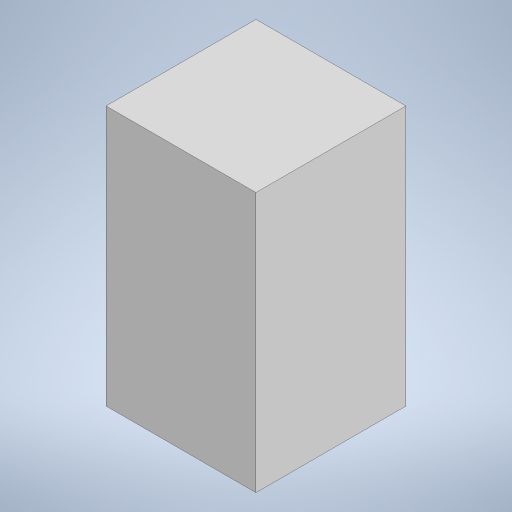
# Autodesk Inventor part: body_luggage
Saved by Autodesk Inventor 2024.3 (Build 283343000, 343)
## iProperties
Created: 2025-04-01
Part Number: body_luggage
Material: 一般
Document SubType Name: Modeling
Designer: yuu53
Density: 1 g/cm^3
Appearance: 既定
Author: yuu53
Autodesk Inventor part; units mm, degrees
ref_plane "YZ Plane" through (0, 0, 0) normal (1, 0, 0) x (0, 1, 0)
ref_plane "XZ Plane" through (0, 0, 0) normal (0, 1, 0) x (-1, 0, 0)
ref_plane "XY Plane" through (0, 0, 0) normal (0, 0, 1) x (1, 0, 0)
sketch "スケッチ1" plane through (0, 0, 0) normal (0, 0, 1) x (1, 0, 0)
  line L0 (-75, -130) -> (75, -130)
  line L1 (75, -130) -> (75, 130)
  line L2 (75, 130) -> (-75, 130)
  line L3 (-75, 130) -> (-75, -130)
  point P0 (0, 0)
  point P1 (75, 0)
  dimension "d0" = 260
  dimension "d1" = 150
  dimension "d3" = 75
  dimension "d4" = 130
  constraints: 8 end point, 2 parallel, 1 horizontal, 1 midpoint, 1 perpendicular
  measures "d0" distance of L0.end L1.end
  measures "d1" distance of L1.end L2.end
  measures "d3" distance from line of L1 point (0, 0)
  measures "d4" distance from line of point (0, 0) L2
extrude "押し出し1" add sketch "スケッチ1" along normal mid plane 150
